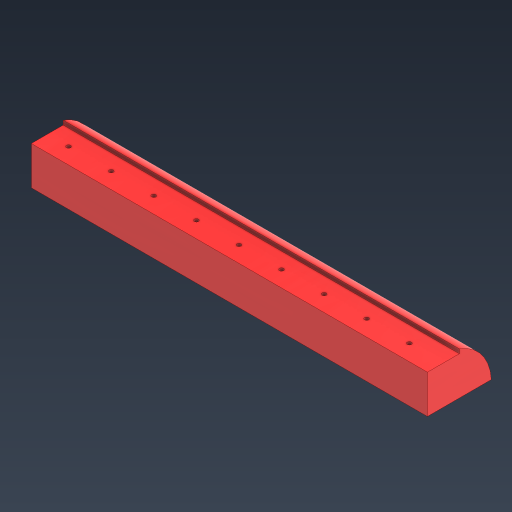
# Autodesk Inventor part: Край задней части корпуса
Saved by Autodesk Inventor 2023.2 (Build 272271030, 271C)
## iProperties
Created: 2025-04-24
Part Number: Край задней части корпуса
Material: Типовые
Document SubType Name: Modeling
Designer: Коноваленко
Density: 1 g/cm^3
Appearance: Светло-красный
Author: Коноваленко
Autodesk Inventor part; units mm, degrees
ref_plane "YZ Plane" through (0, 0, 0) normal (1, 0, 0) x (0, 1, 0)
ref_plane "XZ Plane" through (0, 0, 0) normal (0, 1, 0) x (-1, 0, 0)
ref_plane "XY Plane" through (0, 0, 0) normal (0, 0, 1) x (1, 0, 0)
sketch "Эскиз1" plane through (0, 0, 0) normal (1, 0, 0) x (0, 1, 0)
  line L0 (-8.3221, -14.9171) -> (-8.3221, 15.0829)
  line L1 (-8.3221, 15.0829) -> (31.6779, 15.0829)
  arc A0 (-8.3221, -14.9171) -> (31.6779, 15.0829) centre (-10.7721, 30.0161) ccw
  point P0 (0, 0)
  dimension "d0" = 30
  dimension "d1" = 40
  dimension "d5" = 45
  constraints: 4 end point, 2 point on circle, 1 centre point, 1 horizontal, 1 vertical
  measures "d0" distance of L0.start L0.end
  measures "d1" distance of L0.end L1.end
  measures "d5" radius of A0
extrude "Выдавливание1" add sketch "Эскиз1" along normal mid plane 372
sketch "Эскиз3" plane through (-186, -8.3221, 15.0829) normal (0, 0, 1) x (1, 0, 0)
  line L0 (0, 0) -> (372, 0) projected
  line L1 (372, 40) -> (372, 0) projected
  line L2 (372, 40) -> (0, 40) projected
  line L3 (0, 0) -> (0, 40) projected
  point P0 (186, 8.3221)
extrude "Выдавливание2" add sketch "Эскиз3" along normal blind 30
sketch "Эскиз4" plane through (-186, 31.6779, 15.0829) normal (0, 1, 0) x (1, 0, 0)
  line L0 (372, 0) -> (0, 0) projected
  line L1 (0, 0) -> (0, -30) projected
  line L2 (372, -30) -> (0, -30) projected
  line L3 (372, 0) -> (372, -30) projected
  point P0 (186, 15.0829)
extrude "Выдавливание3" cut sketch "Эскиз4" against normal blind 4
sketch "Эскиз5" plane through (-186, 27.6779, 15.0829) normal (0, 1, 0) x (1, 0, 0)
  line L0 (0, 30) -> (0, -30) projected
  line L1 (0, -15) -> (372, -15) construction
  line L2 (372, 0) -> (372, -30) projected
  circle A0 centre (20, -15) radius 2
  circle A1 centre (60, -15) radius 2
  circle A2 centre (100, -15) radius 2
  circle A3 centre (140, -15) radius 2
  circle A4 centre (180, -15) radius 2
  circle A5 centre (220, -15) radius 2
  circle A6 centre (260, -15) radius 2
  circle A7 centre (300, -15) radius 2
  circle A8 centre (340, -15) radius 2
  circle A9 centre (380, -15) radius 2
  point P0 (186, 15.0829)
  dimension "d10" = 4
  dimension "d11" = 20
  dimension "d14" = 40
  constraints: 10 centre point, 2 end point, 2 horizontal, 2 point on line, 1 midpoint, 18 other
  measures "d10" diameter of A0
  measures "d11" distance from line of L0 A0.centre
  measures "d14" distance of A0.centre A1.centre
extrude "Выдавливание4" cut sketch "Эскиз5" against normal up to surface (36 mm away)
sketch "Эскиз6" plane through (-186, 27.6779, 15.0829) normal (0, 1, 0) x (1, 0, 0)
  line L0 (0, 30) -> (0, -30) projected
  line L1 (0, -14.536) -> (200.0528, -14.536) construction
  line L2 (372, 0) -> (0, 0) projected
  circle A0 centre (10.061, -14.536) radius 8.0645
  circle A1 centre (37.061, -14.536) radius 8.0645
  circle A2 centre (64.061, -14.536) radius 8.0645
  circle A3 centre (91.061, -14.536) radius 8.0645
  circle A4 centre (118.061, -14.536) radius 8.0645
  circle A5 centre (145.061, -14.536) radius 8.0645
  circle A6 centre (172.061, -14.536) radius 8.0645
  point P0 (186, 15.0829)
  dimension "d21" = 14.536
  dimension "d22" = 16.129
  dimension "d23" = 10.061
  dimension "d26" = 27
  constraints: 7 centre point, 2 end point, 2 horizontal, 2 point on line, 12 other
  measures "d21" distance between parallel lines of L2 L1
  measures "d22" diameter of A0
  measures "d23" distance from line of L0 A0.centre
  measures "d26" distance of A0.centre A1.centre
extrude "Выдавливание5" [suppressed]
sketch "Эскиз8" plane through (-186, -8.3221, -14.9171) normal (0, -1, 0) x (1, 0, 0)
  line L0 (372, 40) -> (382, 45)
  line L1 (382, 45) -> (382, 25)
  line L2 (382, 25) -> (372, 30)
  line L3 (372, 0) -> (372, 60) projected
  point P0 (186, 14.9171)
  point P1 (382, 35)
  dimension "d33" = 20
  dimension "d34" = 10
  dimension "d35" = 20
  dimension "d36" = 15
  dimension "d37" = 10
  constraints: 6 end point, 2 midpoint, 1 point on line, 1 vertical
  measures "d33" distance of L0.end L1.end
  measures "d34" distance of L2.end L0.start
  measures "d35" distance of L3.end L0.start
  measures "d36" vertical distance of L3.end L0.end
  measures "d37" distance from line of point (382, 35) L3
extrude "Выдавливание6" [suppressed]
sketch "Эскиз9" plane through (-186, -8.3221, -14.9171) normal (0, -1, 0) x (1, 0, 0)
  line L0 (210, 40) -> (220, 45)
  line L1 (220, 45) -> (220, 25)
  line L2 (220, 25) -> (210, 30)
  line L3 (372, 0) -> (372, 60) projected
  line L4 (-10, 25) -> (-10, 45)
  line L5 (-10, 45) -> (0, 40)
  line L6 (0, 30) -> (-10, 25)
  line L7 (0, 0) -> (0, 60) projected
  point P0 (186, 14.9171)
  point P1 (372, 60)
  constraints: 12 end point, 2 vertical, 13 other
extrude "Выдавливание7" [suppressed]
sketch "Эскиз10" plane through (-186, -8.3221, -14.9171) normal (0, -1, 0) x (1, 0, 0)
  line L0 (-10, 45) -> (0, 40)
  line L1 (-10, 25) -> (-10, 45)
  line L2 (0, 30) -> (-10, 25)
  line L3 (0, 0) -> (0, 60) projected
  point P0 (186, 14.9171)
  constraints: 6 end point, 1 vertical, 6 other
extrude "Выдавливание8" add sketch "Эскиз10" against normal blind 20
sketch "Эскиз11" plane through (-186, -8.3221, -14.9171) normal (0, -1, 0) x (1, 0, 0)
  line L0 (0, 60) -> (372, 60) projected
  line L1 (0, 0) -> (372, 0) projected
  line L2 (0, 30) -> (372, 30) projected
  point P0 (186, 14.9171)
feature "Разделение1" [suppressed]
sketch "Эскиз12" plane through (-186, 27.6779, 15.0829) normal (0, 1, 0) x (1, 0, 0)
  line L0 (0, 0) -> (372, 0) projected
  line L1 (206.541, 0) -> (206.541, -5)
  line L2 (206.541, -5) -> (222.717, -4.95)
  line L3 (222.717, -4.95) -> (222.717, -17.926)
  line L4 (222.717, -17.926) -> (206.541, -20.945)
  line L5 (206.541, -20.945) -> (206.541, -30)
  line L6 (0, -30) -> (372, -30) projected
  line L7 (186, 42) -> (186, -42) projected
  point P0 (186, 15.0829)
  dimension "d54" = 20.541
  dimension "d55" = 16.176
  dimension "d56" = 12.074
  dimension "d57" = 4.95
  dimension "d58" = 9.055
  dimension "d59" = 5
  constraints: 10 end point, 4 point on line, 1 parallel, 1 perpendicular
  measures "d54" distance between parallel lines of L7 L5
  measures "d55" distance between parallel lines of L1 L3
  measures "d56" distance from line of L6 L3.end
  measures "d57" distance from line of L0 L2.end
  measures "d58" distance of L4.end L5.end
  measures "d59" distance of L1.start L1.end
feature "Разделение2" [suppressed]
